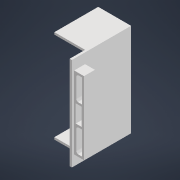
# Autodesk Inventor part: drzalo_vezja
Saved by Autodesk Inventor 2022 (Build 260153000, 153)
## iProperties
Created: 2022-01-23
Part Number: drzalo_vezja
Material: Generic
Document SubType Name: Modeling
Designer: simon
Density: 1 g/cm^3
Appearance: Default
Author: simon
Autodesk Inventor part; units mm, degrees
ref_plane "YZ Plane" through (0, 0, 0) normal (1, 0, 0) x (0, 1, 0)
ref_plane "XZ Plane" through (0, 0, 0) normal (0, 1, 0) x (-1, 0, 0)
ref_plane "XY Plane" through (0, 0, 0) normal (0, 0, 1) x (1, 0, 0)
sketch "Sketch1" plane through (0, 0, 0) normal (0, 0, 1) x (1, 0, 0)
  arc A0 (-0.5, 10.6) -> (-2.5, 8.6) centre (-0.5, 8.6) ccw projected
  line L0 (-2.5, 8.6) -> (-2.5, -8.6) projected
  arc A1 (-2.5, -8.6) -> (-0.5, -10.6) centre (-0.5, -8.6) ccw projected
  line L1 (-0.5, -10.6) -> (2.5, -10.6) projected
  line L2 (2.5, -10.6) -> (2.5, 10.6) projected
  line L3 (2.5, 10.6) -> (-0.5, 10.6) projected
  line L4 (2.5, -51.8) -> (10.3, -51.8) projected
  arc A2 (10.3, -51.8) -> (12.3, -49.8) centre (10.3, -49.8) ccw projected
  line L5 (12.3, -49.8) -> (12.3, -43.8) projected
  arc A3 (14.3, -41.8) -> (12.3, -43.8) centre (14.3, -43.8) ccw projected
  line L6 (14.3, -41.8) -> (33.1, -41.8) projected
  arc A4 (35.1, -43.8) -> (33.1, -41.8) centre (33.1, -43.8) ccw projected
  line L7 (35.1, -43.8) -> (35.1, -49.8) projected
  arc A5 (35.1, -49.8) -> (37.1, -51.8) centre (37.1, -49.8) ccw projected
  line L8 (37.1, -51.8) -> (47.9, -51.8) projected
  arc A6 (47.9, -51.8) -> (49.9, -49.8) centre (47.9, -49.8) ccw projected
  line L9 (49.9, -49.8) -> (49.9, -27.6) projected
  arc A7 (51.9, -25.6) -> (49.9, -27.6) centre (51.9, -27.6) ccw projected
  line L10 (51.9, -25.6) -> (137.9, -25.6) projected
  arc A8 (139.9, -27.6) -> (137.9, -25.6) centre (137.9, -27.6) ccw projected
  line L11 (139.9, -27.6) -> (139.9, -49.8) projected
  arc A9 (139.9, -49.8) -> (141.9, -51.8) centre (141.9, -49.8) ccw projected
  line L12 (141.9, -51.8) -> (154.1, -51.8) projected
  arc A10 (154.1, -51.8) -> (156.1, -49.8) centre (154.1, -49.8) ccw projected
  line L13 (156.1, -49.8) -> (156.1, -41.8) projected
  line L14 (156.1, -41.8) -> (176.1, -41.8) projected
  line L15 (176.1, -41.8) -> (176.1, -49.8) projected
  arc A11 (176.1, -49.8) -> (178.1, -51.8) centre (178.1, -49.8) ccw projected
  line L16 (178.1, -51.8) -> (190.3, -51.8) projected
  arc A12 (190.3, -51.8) -> (192.3, -49.8) centre (190.3, -49.8) ccw projected
  line L17 (192.3, -49.8) -> (192.3, -38.8) projected
  arc A13 (192.3, -38.8) -> (190.3, -36.8) centre (190.3, -38.8) ccw projected
  line L18 (190.3, -36.8) -> (189.3, -36.8) projected
  arc A14 (187.3, -34.8) -> (189.3, -36.8) centre (189.3, -34.8) ccw projected
  line L19 (187.3, -34.8) -> (187.3, -6.4) projected
  arc A15 (189.3, -4.4) -> (187.3, -6.4) centre (189.3, -6.4) ccw projected
  line L20 (189.3, -4.4) -> (190.3, -4.4) projected
  arc A16 (190.3, -4.4) -> (192.3, -2.4) centre (190.3, -2.4) ccw projected
  line L21 (192.3, -2.4) -> (192.3, 8.6) projected
  arc A17 (192.3, 8.6) -> (190.3, 10.6) centre (190.3, 8.6) ccw projected
  line L22 (190.3, 10.6) -> (178.1, 10.6) projected
  arc A18 (178.1, 10.6) -> (176.1, 8.6) centre (178.1, 8.6) ccw projected
  line L23 (176.1, 8.6) -> (176.1, 2.6) projected
  arc A19 (174.1, 0.6) -> (176.1, 2.6) centre (174.1, 2.6) ccw projected
  line L24 (174.1, 0.6) -> (158.1, 0.6) projected
  arc A20 (156.1, 2.6) -> (158.1, 0.6) centre (158.1, 2.6) ccw projected
  line L25 (156.1, 2.6) -> (156.1, 8.6) projected
  arc A21 (156.1, 8.6) -> (154.1, 10.6) centre (154.1, 8.6) ccw projected
  line L26 (154.1, 10.6) -> (141.9, 10.6) projected
  arc A22 (141.9, 10.6) -> (139.9, 8.6) centre (141.9, 8.6) ccw projected
  line L27 (139.9, 8.6) -> (139.9, -13.6) projected
  arc A23 (137.9, -15.6) -> (139.9, -13.6) centre (137.9, -13.6) ccw projected
  line L28 (51.9, -15.6) -> (137.9, -15.6) projected
  arc A24 (49.9, -13.6) -> (51.9, -15.6) centre (51.9, -13.6) ccw projected
  line L29 (49.9, -13.6) -> (49.9, 8.6) projected
  arc A25 (49.9, 8.6) -> (47.9, 10.6) centre (47.9, 8.6) ccw projected
  line L30 (47.9, 10.6) -> (37.1745, 10.6) projected
  arc A26 (37.1745, 10.6) -> (35.1745, 8.6) centre (37.1745, 8.6) ccw projected
  line L31 (35.1745, 8.6) -> (35.1745, 2.6) projected
  arc A27 (33.1745, 0.6) -> (35.1745, 2.6) centre (33.1745, 2.6) ccw projected
  line L32 (33.1745, 0.6) -> (14.3, 0.6) projected
  arc A28 (12.3, 2.6) -> (14.3, 0.6) centre (14.3, 2.6) ccw projected
  line L33 (12.3, 2.6) -> (12.3, 8.6) projected
  arc A29 (12.3, 8.6) -> (10.3, 10.6) centre (10.3, 8.6) ccw projected
  line L34 (10.3, 10.6) -> (2.5, 10.6) projected
  line L35 (2.5, 10.6) -> (2.5, -51.8) projected
  circle A30 centre (181.65, 5.6) radius 1.25 projected
  circle A31 centre (181.65, -46.8) radius 1.25 projected
  circle A32 centre (150.55, -46.8) radius 1.25 projected
  circle A33 centre (166.1, -20.6) radius 12.5 projected
  circle A34 centre (150.55, 5.6) radius 1.25 projected
  circle A35 centre (39.25, -46.8) radius 1.25 projected
  circle A36 centre (8.15, 5.6) radius 1.25 projected
  circle A37 centre (8.15, -46.8) radius 1.25 projected
  circle A38 centre (23.7, -20.6) radius 12.5 projected
  circle A39 centre (39.25, 5.6) radius 1.25 projected
  arc A40 (-0.5, -30.6) -> (-2.5, -32.6) centre (-0.5, -32.6) ccw projected
  line L36 (-2.5, -32.6) -> (-2.5, -49.8) projected
  arc A41 (-2.5, -49.8) -> (-0.5, -51.8) centre (-0.5, -49.8) ccw projected
  line L37 (-0.5, -51.8) -> (2.5, -51.8) projected
  line L38 (2.5, -51.8) -> (2.5, -30.6) projected
  line L39 (2.5, -30.6) -> (-0.5, -30.6) projected
  arc A42 (-0.5, 12.6) -> (-4.5, 8.6) centre (-0.5, 8.6) ccw
  line L40 (-4.5, 8.6) -> (-4.5, -8.6)
  arc A43 (-4.5, -8.6) -> (-0.5, -12.6) centre (-0.5, -8.6) ccw
  line L41 (-0.5, -12.6) -> (4.5, -12.6)
  line L42 (4.5, -12.6) -> (4.5, 12.6)
  line L43 (4.5, 12.6) -> (-0.5, 12.6)
  arc A44 (-0.5, -28.6) -> (-4.5, -32.6) centre (-0.5, -32.6) ccw
  line L44 (-0.5, -28.6) -> (4.5, -28.6)
  line L45 (4.5, -28.6) -> (4.5, -53.8)
  line L46 (4.5, -53.8) -> (-0.5, -53.8)
  arc A45 (-4.5, -49.8) -> (-0.5, -53.8) centre (-0.5, -49.8) ccw
  line L47 (-4.5, -49.8) -> (-4.5, -32.6)
  line L48 (4.5, -12.6) -> (4.5, -28.6)
  line L49 (-4.5, -8.6) -> (-4.5, -32.6)
  line L50 (0, -28.6) -> (0, -12.6)
  line L51 (-3, -12.6) -> (3, -12.6)
  line L52 (3, -12.6) -> (3, -28.6)
  line L53 (3, -28.6) -> (-3, -28.6)
  line L54 (-3, -28.6) -> (-3, -12.6)
  line L55 (-3, -12.6) -> (3, -28.6) construction
  line L56 (3, -12.6) -> (-3, -28.6) construction
  arc A46 (-0.5, -30.5065) -> (-2.5935, -32.6) centre (-0.5, -32.6) ccw
  line L57 (-0.5, -30.5065) -> (2.5935, -30.5065)
  line L58 (2.5935, -30.5065) -> (2.5935, -51.8935)
  line L59 (2.5935, -51.8935) -> (-0.5, -51.8935)
  arc A47 (-2.5935, -49.8) -> (-0.5, -51.8935) centre (-0.5, -49.8) ccw
  line L60 (-2.5935, -49.8) -> (-2.5935, -32.6)
  arc A48 (-2.6, -8.6) -> (-0.5, -10.7) centre (-0.5, -8.6) ccw
  line L61 (-2.6, -8.6) -> (-2.6, 8.6)
  arc A49 (-0.5, 10.7) -> (-2.6, 8.6) centre (-0.5, 8.6) ccw
  line L62 (-0.5, 10.7) -> (2.6, 10.7)
  line L63 (2.6, 10.7) -> (2.6, -10.7)
  line L64 (2.6, -10.7) -> (-0.5, -10.7)
  line L65 (2.5, -12.6) -> (2.5, -13.431)
  line L66 (2.5, -13.431) -> (2.5, -15.7904)
  line L67 (2.5, -15.7904) -> (2.5, -28.2258)
  line L68 (2.5, -28.2258) -> (2.5, -28.5718)
  line L69 (2.5, -28.5718) -> (2.5, -28.6211)
  line L70 (4.5, 12.6) -> (-4.5, 12.6)
  line L71 (-4.5, 12.6) -> (-4.5, -53.8)
  line L72 (-4.5, -53.8) -> (4.5, -53.8)
  line L73 (4.5, -53.8) -> (4.5, 12.6)
  point P0 (0, 0)
  point P1 (0, -20.6)
  point P2 (2.5, -12.6)
  point P3 (2.5, -28.6)
  point P4 (2.5935, -51.8)
  point P5 (4.5, -51.8)
  point P6 (2.5, -30.5065)
  point P7 (-0.5, -28.6)
  point P8 (-0.5, -12.6)
  point P9 (2.5, -10.7)
  point P10 (4.5, 10.6)
  point P11 (2.6, 10.6)
  point P12 (-4.5, 8.6)
  point P13 (-0.5, 12.6)
  point P14 (-0.5, -53.8)
  point P15 (-4.5, -49.8)
  dimension "d0" = 2
  dimension "d1" = 2
  dimension "d2" = 6
  dimension "d3" = 0.1
  constraints: 68 end point, 17 point on circle, 8 centre point, 5 parallel, 4 perpendicular, 3 midpoint, 3 point on line, 1 horizontal, 1 tangent, 27 other
  measures "d0" distance between parallel lines of L3 L43
  measures "d1" radial gap between concentric circles of A40 A44
  measures "d2" distance of L51.start L51.end
  measures "d3" radial gap between concentric circles of A1 A48
extrude "Extrusion1" add sketch "Sketch1" along normal blind 10 contours L63 L62 A49 L61 A48 L64 L35 L41 A43 L40 A42 L43 L42 L34 | L34 L42 L41 L35 L64 L63 | L41 L52 L44 L35 | L48 L44 L52 L41 | L45 L4 L58 L57 L35 L44 | A42 L71 L70 | L51 L54 L53 A44 L49 A43 | L44 L35 L57 A46 L60 A47 L59 L58 L4 L45 L46 A45 L47 A44 | L72 L71 A45
sketch "Sketch10" plane through (-4.5, -53.8, 0) normal (-1, 0, 0) x (0, 0, 1)
  line L0 (0, 66.4) -> (0, 0) projected
  line L1 (0, 0) -> (10, 0) projected
  line L2 (10, 66.4) -> (10, 0) projected
  line L3 (0, 66.4) -> (10, 66.4) projected
  line L4 (0, 1.9065) -> (0, 0)
  line L5 (0, -7.3) -> (10, -7.3)
  line L6 (10, -7.3) -> (10, 73.7)
  line L7 (10, 73.7) -> (0, 73.7)
  line L8 (0, 73.7) -> (10, -7.3) construction
  line L9 (0, -7.3) -> (10, 73.7) construction
  line L10 (0, 1.9065) -> (10, 1.9065) projected
  line L11 (0, 73.7) -> (81, 73.7) construction
  line L12 (12, -9.3) -> (-2, -9.3)
  line L13 (-2, -9.3) -> (-2, 75.7)
  line L14 (-2, 75.7) -> (12, 75.7)
  line L15 (12, 75.7) -> (12, -9.3)
  line L16 (0, 73.7) -> (-40, 73.7)
  line L17 (-40, 73.7) -> (-40, -7.3)
  line L18 (-40, -7.3) -> (0, -7.3)
  line L19 (0, 0) -> (0, 1.9065)
  line L20 (-42, 75.7) -> (2, 75.7)
  line L21 (2, -9.3) -> (-42, -9.3)
  line L22 (-42, -9.3) -> (-42, 75.7)
  line L23 (2, -7.3) -> (2, -9.3)
  line L24 (10, -7.3) -> (10, -9.3)
  line L25 (10, 73.7) -> (10, 75.7)
  point P0 (0, 53.8)
  point P1 (5, 33.2)
  point P2 (-2, -9.3)
  point P3 (-2, 73.7)
  point P4 (-2, -9.3)
  point P5 (-2, -7.3)
  dimension "d64" = 81
  dimension "d65" = 90
  dimension "d66" = 2
  dimension "d67" = 40
  dimension "d68" = 2
  constraints: 42 end point, 8 parallel, 6 point on line, 5 perpendicular, 2 horizontal, 2 midpoint, 1 vertical, 2 other
  measures "d64" distance of L7.end L5.start
  measures "d65" angle of L4 L11
  measures "d66" distance between parallel lines of L5 L12
  measures "d67" distance of L18.end L17.end
  measures "d68" distance between parallel lines of L16 L20
extrude "Extrusion9" add sketch "Sketch10" along normal blind 2
extrude "Extrusion10" add sketch "Sketch10" along normal blind 30 contours L16 L17 L18 L13 L21 L22 L20
body "Solid1"
